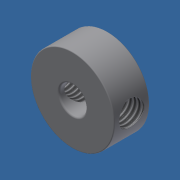
# Autodesk Inventor part: Smiglo-tuleja trzymajaca
Saved by Autodesk Inventor 2014 SP1 (Build 180222100, 222)
## iProperties
Created: 2014-09-01
Part Number: Smiglo-tuleja trzymajaca
Material: Ogólny
Document SubType Name: Modeling
Designer: Marcin
Density: 1 g/cm^3
Appearance: Domyślna
Author: Marcin
Autodesk Inventor part; units mm, degrees
ref_plane "XZ Plane" through (0, 0, 0) normal (0, 1, 0) x (-1, 0, 0)
ref_plane "XY Plane" through (0, 0, 0) normal (0, 0, 1) x (1, 0, 0)
sketch "Szkic1" plane through (0, 0, 0) normal (0, 1, 0) x (-1, 0, 0)
  circle A0 centre (0, 0) radius 4.75
  circle A1 centre (0, 0) radius 1.5
  dimension "d0" = 9.5
  dimension "d1" = 3
  constraints: 2 centre point, 2 coincident
  measures "d0" diameter of A0
  measures "d1" diameter of A1
extrude "Wyciągnięcie proste1" add sketch "Szkic1" along normal blind 4
ref_plane "Płaszczyzna konstrukcyjna1" through (4.75, 0, 0) normal (1, 0, 0) x (0, 1, 0)
sketch "Szkic2" plane through (4.75, 0, 0) normal (1, 0, 0) x (0, 1, 0)
  line L0 (-0.6, 0) -> (3.6, 0) projected
  line L1 (4, -4.75) -> (4, 4.75) projected
  line L2 (0, 4.75) -> (0, -4.75) projected
  circle A0 centre (2, 0) radius 1.4
  line L3 (2, 0) -> (4, 0)
  line L4 (2, 0) -> (0, 0)
  dimension "d5" = 2.8
  constraints: 4 end point, 2 collinear, 1 centre point, 1 midpoint, 1 point on line
  measures "d5" diameter of A0
hole "Otwór1" at (4.75, 2, 0) direction (-1, 0, 0) diameter 2.8 end through all
thread "Gwint1" size "M3x0.5" class "6H" standard "ANSI Metric M Profile" full length
thread "Gwint2" size "M3x0.5" class "6H" standard "ANSI Metric M Profile" full length
fillet "Zaokrąglenie1" radius 0.1 2 edges at (4.75, 4, 0) (4.75, 0, 0)
fillet "Zaokrąglenie2" radius 0.2 1 edges at (1.5, 4, 0)
fillet "Zaokrąglenie3" radius 0.2 1 edges at (1.5, 0, 0)
fillet "Zaokrąglenie4" radius 0.05 6 edges at (-4.6327, 1.0728, -1.049) (-4.539, 1.9999, 1.4) (-4.6327, 2.9272, -1.0489) (4.6327, 1.0728, -1.049) (4.6327, 2.9272, -1.0489) (4.539, 1.9999, 1.4)
fillet_without_effect "Zaokrąglenie5"
equation "\"d6\" = d5"
equation "\"d4\" = 0.5 * d0"
